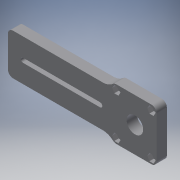
# Autodesk Inventor part: Bearing_support_inside
Saved by Autodesk Inventor 2019.3 (Build 233278000, 278)
## iProperties
Created: 2020-08-25
Part Number: Bearing_support_inside
Material: Generisch
Document SubType Name: Modeling
Designer: Nicolas Frick
Density: 1 g/cm^3
Appearance: Vorgabe
Author: Nicolas Frick
Autodesk Inventor part; units mm, degrees
ref_plane "YZ Plane" through (0, 0, 0) normal (1, 0, 0) x (0, 1, 0)
ref_plane "XZ Plane" through (0, 0, 0) normal (0, 1, 0) x (-1, 0, 0)
ref_plane "XY Plane" through (0, 0, 0) normal (0, 0, 1) x (1, 0, 0)
sketch "Skizze1" plane through (0, 0, 0) normal (0, 0, 1) x (1, 0, 0)
  circle A0 centre (2.19, 20) radius 2 projected
  circle A1 centre (-31.81, 20) radius 2 projected
  arc A2 (-31.81, 25) -> (-36.81, 20) centre (-31.81, 20) ccw projected
  line L0 (-36.81, 20) -> (-36.81, 16) projected
  line L1 (7.19, 16) -> (7.19, 20) projected
  arc A3 (7.19, 20) -> (2.19, 25) centre (2.19, 20) ccw projected
  line L2 (2.19, 25) -> (-31.81, 25) projected
  circle A4 centre (2.19, -20) radius 2 projected
  circle A5 centre (-31.81, -20) radius 2 projected
  arc A6 (-36.81, -20) -> (-31.81, -25) centre (-31.81, -20) ccw projected
  line L3 (-31.81, -25) -> (2.19, -25) projected
  arc A7 (2.19, -25) -> (7.19, -20) centre (2.19, -20) ccw projected
  line L4 (7.19, -20) -> (7.19, -16) projected
  line L5 (-36.81, -16) -> (-36.81, -20) projected
  line L6 (-29.81, -10) -> (-36.81, -10) projected
  line L7 (-36.81, -16) -> (-36.81, -10) projected
  line L8 (7.19, 16) -> (7.19, -16) projected
  line L9 (-36.81, 10) -> (-36.81, 16) projected
  line L10 (-36.81, 10) -> (-29.81, 10) projected
  line L11 (-29.81, 10) -> (-29.81, -10) projected
  circle A8 centre (-13.81, 0) radius 8 projected
  point P0 (0, 0)
extrude "Extrusion1" add sketch "Skizze1" along normal blind 10
sketch "Skizze3" plane through (-36.81, 10, 0) normal (-1, 0, 0) x (0, 0, 1)
  line L0 (0, 10) -> (0, 0) projected
  line L1 (0, 0) -> (10, 0) projected
  line L2 (10, 10) -> (10, 0) projected
  line L3 (0, 10) -> (10, 10) projected
  line L4 (0, -20) -> (0, -30) projected
  line L5 (0, -30) -> (10, -30) projected
  line L6 (10, -20) -> (10, -30) projected
  line L7 (0, -20) -> (10, -20) projected
  line L8 (10, -0.1675) -> (10, -20.1669) projected
  line L9 (0, 0) -> (0, -20) projected
  line L10 (10, -35) -> (10, -30) projected
  line L11 (0, 10) -> (10, 10)
  line L12 (10, 10) -> (10, -30)
  line L13 (10, -30) -> (0, -30)
  line L14 (0, -30) -> (0, 10)
  point P0 (0, -10)
  constraints: 8 end point, 2 parallel, 1 horizontal, 1 perpendicular
extrude "Extrusion3" add sketch "Skizze3" along normal blind 100
sketch "Skizze4" plane through (0, 0, 10) normal (0, 0, 1) x (1, 0, 0)
  line L0 (-36.81, 20) -> (-136.81, 20) projected
  arc A0 (-31.81, 25) -> (-36.81, 20) centre (-31.81, 20) ccw projected
  line L1 (-36.81, 20) -> (-136.81, 20) projected
  arc A1 (-31.81, 25) -> (-36.81, 20) centre (-31.81, 20) ccw projected
  arc A2 (-45.8607, 20) -> (-35.3455, 23.5355) centre (-45.0384, 34.959) ccw
  line L2 (-44.2162, 20) -> (-36.81, 20)
  arc A3 (-35.3455, 23.5355) -> (-36.81, 20) centre (-31.81, 20) ccw
  line L3 (-45.8607, 0) -> (-28.5304, 0)
  line L4 (-36.81, -20) -> (-136.81, -20)
  arc A4 (-36.81, -20) -> (-31.81, -25) centre (-31.81, -20) ccw
  arc A5 (-35.3455, -23.5355) -> (-45.8607, -20) centre (-45.0384, -34.959) ccw
  line L5 (-36.81, -20) -> (-136.81, -20) projected
  line L6 (-44.2159, -20) -> (-36.81, -20)
  arc A6 (-36.81, -20) -> (-31.81, -25) centre (-31.81, -20) ccw projected
  arc A7 (-36.81, -20) -> (-31.81, -25) centre (-31.81, -20) ccw
  arc A8 (-35.1548, -23.7165) -> (-45.8607, -20) centre (-44.9788, -34.7378) ccw
  point P0 (0, 0)
  constraints: 19 point on circle, 8 end point, 7 symmetric about line, 6 centre point, 3 point on line, 2 collinear, 2 concentric, 1 horizontal, 2 other
extrude "Extrusion4" add sketch "Skizze4" against normal blind 10 contours L0 A2 A0 | L4 A4 A5 A8
fillet "Rundung1" radius 5 2 edges at (-136.81, 20, 5) (-136.81, -20, 5)
sketch "Skizze10" plane through (0, 0, 0) normal (0, 0, -1) x (-1, 0, 0)
  line L0 (36.8821, 9.8325) -> (29.8823, 9.8834) construction
  line L1 (29.7369, -10.116) -> (36.7367, -10.1669) construction
  line L2 (36.81, 10) -> (29.81, 10) projected
  line L3 (29.81, -10) -> (36.81, -10) projected
  line L4 (136.81, 15) -> (136.81, -15) projected
  line L5 (36.81, 10) -> (136.81, 10)
  line L6 (136.81, 10) -> (136.81, -10)
  line L7 (136.81, -10) -> (36.81, -10)
  line L8 (36.81, -10) -> (36.81, 10)
  point P0 (0, 0)
  constraints: 8 end point, 2 parallel, 1 horizontal, 1 perpendicular, 1 point on line
extrude "Extrusion10" add sketch "Skizze10" along normal blind 5
fillet "Rundung3" radius 5 2 edges at (-136.81, 10, -2.5) (-136.81, -10, -2.5)
sketch "Skizze11" plane through (0, 0, -5) normal (0, 0, -1) x (-1, 0, 0)
  line L0 (131.81, 10) -> (36.81, 10) construction
  line L1 (36.81, -10) -> (131.81, -10) construction
  line L2 (40.8, 0) -> (128.9956, 0) construction
  line L3 (45.4, -4.6) -> (124.3956, -4.6)
  line L4 (124.3956, 4.6) -> (45.4, 4.6)
  arc A0 (45.4, 4.6) -> (45.4, -4.6) centre (45.4, 0) ccw
  arc A1 (124.3956, -4.6) -> (124.3956, 4.6) centre (124.3956, 0) ccw
  point P0 (0, 0)
  point P1 (84.8978, 0)
  dimension "d40" = 9.2
  constraints: 8 end point, 6 point on circle, 4 tangent, 2 centre point, 2 point on line, 1 horizontal, 1 midpoint, 1 parallel
  measures "d40" diameter of A1
extrude "Extrusion11" cut sketch "Skizze11" against normal blind 4.2
sketch "Skizze12" plane through (0, 0, -0.8) normal (0, 0, -1) x (-1, 0, 0)
  line L0 (124.3956, -4.6) -> (45.4, -4.6) projected
  arc A0 (124.3956, -4.6) -> (124.3956, 4.6) centre (124.3956, 0) ccw projected
  line L1 (45.4, 4.6) -> (124.3956, 4.6) projected
  arc A1 (45.4, 4.6) -> (45.4, -4.6) centre (45.4, 0) ccw projected
  line L2 (45.4, 0) -> (124.3956, 0) construction
  line L3 (47.55, -2.15) -> (122.2456, -2.15)
  line L4 (122.2456, 2.15) -> (47.55, 2.15)
  arc A2 (47.55, 2.15) -> (47.55, -2.15) centre (47.55, 0) ccw
  arc A3 (122.2456, -2.15) -> (122.2456, 2.15) centre (122.2456, 0) ccw
  point P0 (0, 0)
  point P1 (84.8978, 0)
  dimension "d43" = 4.3
  constraints: 8 end point, 6 point on circle, 4 tangent, 2 centre point, 2 point on line, 1 horizontal, 1 midpoint, 1 parallel
  measures "d43" diameter of A3
extrude "Extrusion12" cut sketch "Skizze12" against normal through all contours A2 L4 A3 L3
sketch "Skizze13" plane through (0, 0, 10) normal (0, 0, 1) x (1, 0, 0)
  circle A0 centre (-31.81, 20) radius 2 construction
  circle A1 centre (2.19, 20) radius 2 construction
  circle A2 centre (2.19, -20) radius 2 construction
  circle A3 centre (-31.81, -20) radius 2 construction
  line L0 (-31.81, 20) -> (2.19, 20) construction
  line L1 (2.19, 20) -> (2.19, -20) construction
  line L2 (-31.81, 20) -> (-31.81, 23.5) construction
  line L3 (-31.81, 23.5) -> (-29.9614, 23.5)
  line L4 (-29.9614, 23.5) -> (-33.1306, 23.5)
  line L5 (-29.81, 23.5) -> (-27.7789, 20.0179)
  line L6 (-27.7789, 20.0179) -> (-29.7789, 16.5179)
  line L7 (-29.7789, 16.5179) -> (-33.81, 16.5)
  line L8 (-33.81, 16.5) -> (-35.8411, 19.9821)
  line L9 (-35.8411, 19.9821) -> (-33.8411, 23.4821)
  line L10 (-33.8411, 23.4821) -> (-29.81, 23.5)
  line L11 (2.19, 20) -> (2.19, 23.5) construction
  line L12 (2.19, 23.5) -> (4.0386, 23.5)
  line L13 (4.0386, 23.5) -> (0.8694, 23.5)
  line L14 (4.19, 23.5) -> (6.2211, 20.0179)
  line L15 (6.2211, 20.0179) -> (4.2211, 16.5179)
  line L16 (4.2211, 16.5179) -> (0.19, 16.5)
  line L17 (0.19, 16.5) -> (-1.8411, 19.9821)
  line L18 (-1.8411, 19.9821) -> (0.1589, 23.4821)
  line L19 (0.1589, 23.4821) -> (4.19, 23.5)
  line L20 (-31.81, -20) -> (-31.81, -16.5) construction
  line L21 (-31.81, -16.5) -> (-29.9614, -16.5)
  line L22 (-29.9614, -16.5) -> (-33.1306, -16.5)
  line L23 (-29.81, -16.5) -> (-27.7789, -19.9821)
  line L24 (-27.7789, -19.9821) -> (-29.7789, -23.4821)
  line L25 (-29.7789, -23.4821) -> (-33.81, -23.5)
  line L26 (-33.81, -23.5) -> (-35.8411, -20.0179)
  line L27 (-35.8411, -20.0179) -> (-33.8411, -16.5179)
  line L28 (-33.8411, -16.5179) -> (-29.81, -16.5)
  line L29 (2.19, -20) -> (2.19, -16.5) construction
  line L30 (2.19, -16.5) -> (4.0386, -16.5)
  line L31 (4.0386, -16.5) -> (0.8694, -16.5)
  line L32 (4.19, -16.5) -> (6.2211, -19.9821)
  line L33 (6.2211, -19.9821) -> (4.2211, -23.4821)
  line L34 (4.2211, -23.4821) -> (0.19, -23.5)
  line L35 (0.19, -23.5) -> (-1.8411, -20.0179)
  line L36 (-1.8411, -20.0179) -> (0.1589, -16.5179)
  line L37 (0.1589, -16.5179) -> (4.19, -16.5)
  point P0 (0, 0)
  dimension "d61" = 3.5
  dimension "d64" = 34
  dimension "d67" = 40
  constraints: 76 end point, 4 coincident, 4 point on line, 3 horizontal, 1 vertical, 74 other
  measures "d61" distance of L0.start L2.end
  measures "d64" distance of L0.start L11.start
  measures "d67" distance of L0.start L20.start
extrude "Extrusion14" cut sketch "Skizze13" against normal blind 4.3
sketch "Skizze14" plane through (0, 0, 0) normal (0, 0, -1) x (-1, 0, 0)
  line L0 (29.81, 10) -> (29.81, -10) projected
  line L1 (36.81, 10) -> (29.81, 10) projected
  line L2 (36.81, -16.5129) -> (36.81, 16.5129) projected
  line L3 (29.81, -10) -> (36.81, -10) projected
  point P0 (0, 0)
extrude "Extrusion15" add sketch "Skizze14" against normal up to surface (10 mm away)
